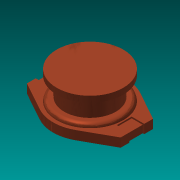
# Autodesk Inventor part: SDR1005
Saved by Autodesk Inventor 2015 (Build 190159000, 159)
## iProperties
Created: 2014-10-16
Part Number: SDR1005
Material: Generic
Document SubType Name: Modeling
Designer: Sawaiz Syed
Density: 1 g/cm^3
Appearance: Copper - Satin
Author: Sawaiz Syed
Autodesk Inventor part; units mm, degrees
ref_plane "YZ Plane" through (0, 0, 0) normal (1, 0, 0) x (0, 1, 0)
ref_plane "XZ Plane" through (0, 0, 0) normal (0, 1, 0) x (-1, 0, 0)
ref_plane "XY Plane" through (0, 0, 0) normal (0, 0, 1) x (1, 0, 0)
sketch "Sketch1" plane through (0, 0, 0) normal (0, 0, 1) x (1, 0, 0)
  line L0 (-6.35, 5) -> (6.35, 5)
  line L1 (6.35, 5) -> (6.35, -5)
  line L2 (6.35, -5) -> (-6.35, -5)
  line L3 (-6.35, -5) -> (-6.35, 5)
  line L4 (-6.35, 5) -> (6.35, -5) construction
  line L5 (6.35, 5) -> (-6.35, -5) construction
  line L6 (-2.4214, 4.3746) -> (-6.35, 2.2)
  line L7 (-2.4214, -4.3746) -> (-6.35, -2.2)
  line L8 (0, -5) -> (0, 5)
  line L9 (2.4214, 4.3746) -> (6.35, 2.2)
  line L10 (2.4214, -4.3746) -> (6.35, -2.2)
  line L11 (-6.35, 2.2) -> (-6.35, -2.2)
  line L12 (6.35, -2.2) -> (6.35, 2.2)
  arc A0 (-2.4214, -4.3746) -> (2.4214, -4.3746) centre (0, 0) ccw
  arc A1 (2.4214, 4.3746) -> (-2.4214, 4.3746) centre (0, 0) ccw
  point P0 (-1.2915, 5)
  point P1 (-1.2915, -5)
  point P2 (1.2915, 5)
  point P3 (1.2915, -5)
  dimension "d0" = 12.7
  dimension "d1" = 10
  dimension "d3" = 2.8
  dimension "d4" = 2.8
  constraints: 26 end point, 6 point on circle, 4 midpoint, 4 point on line, 4 symmetric about line, 3 tangent, 2 centre point, 2 collinear, 2 parallel, 1 coincident, 1 horizontal, 1 perpendicular
  measures "d0" distance of L1.end L2.end
  measures "d1" distance of L0.end L1.end
  measures "d3" distance of L0.start L6.end
  measures "d4" distance of L2.end L7.end
extrude "Extrusion1" add sketch "Sketch1" along normal blind 1.2 contours A1 L9 L1 L10 A0 L8 | L8 A0 L7 L3 L6 A1
sketch "Sketch2" plane through (0, 0, 1.2) normal (0, 0, 1) x (1, 0, 0)
  arc A0 (2.4214, 4.3746) -> (-2.4214, 4.3746) centre (0, 0) ccw projected
  circle A1 centre (0, 0) radius 3.5
  circle A2 centre (0, 0) radius 4.5
  dimension "d7" = 7
  dimension "d8" = 1
  constraints: 2 centre point, 1 coincident
  measures "d7" diameter of A1
  measures "d8" radial gap between concentric circles of A1 A2
extrude "Extrusion2" add sketch "Sketch2" along normal blind 0.5 contours A1 | A2
sketch "Sketch3" plane through (0, 0, 1.7) normal (0, 0, 1) x (1, 0, 0)
  circle A0 centre (0, 0) radius 4.5 projected
  circle A1 centre (0, 0) radius 3.5
  dimension "d11" = 7
  constraints: 1 centre point, 1 coincident
  measures "d11" diameter of A1
extrude "Extrusion3" add sketch "Sketch3" along normal blind 2.5 contours A1
sketch "Sketch4" plane through (0, 0, 4.2) normal (0, 0, 1) x (1, 0, 0)
  circle A0 centre (0, 0) radius 4.5
  dimension "d14" = 9
  constraints: 1 centre point, 1 coincident
  measures "d14" diameter of A0
extrude "Extrusion4" add sketch "Sketch4" along normal blind 0.8
fillet "Fillet1" radius 0.5 1 edges at (-4.5, 0, 1.7)
sketch "Sketch5" plane through (0, 0, 1.2) normal (0, 0, 1) x (1, 0, 0)
  circle A0 centre (0, 0) radius 4.5 projected
  line L0 (-6.35, 2.2) -> (-6.35, -2.2) projected
  line L1 (-6.35, -2.2) -> (-2.4214, -4.3746) projected
  arc A1 (-2.4214, -4.3746) -> (2.4214, -4.3746) centre (0, 0) ccw projected
  line L2 (2.4214, -4.3746) -> (6.35, -2.2) projected
  line L3 (6.35, -2.2) -> (6.35, 2.2) projected
  line L4 (6.35, 2.2) -> (2.4214, 4.3746) projected
  arc A2 (2.4214, 4.3746) -> (-2.4214, 4.3746) centre (0, 0) ccw projected
  line L5 (-2.4214, 4.3746) -> (-6.35, 2.2) projected
  line L6 (-6.35, 2.2) -> (-6.35, -2.2) projected
  line L7 (-6.35, 1) -> (-6.15, 1)
  line L8 (-6.15, 1) -> (-6.15, -1)
  line L9 (-6.15, -1) -> (-6.35, -1)
  line L10 (-6.35, -1) -> (-6.35, 1)
  line L11 (6.35, -1) -> (6.15, -1)
  line L12 (6.15, -1) -> (6.15, 1)
  line L13 (6.15, 1) -> (6.35, 1)
  line L14 (6.35, 1) -> (6.35, -1)
  point P0 (6.35, 0)
  point P1 (-6.35, 0)
  dimension "d18" = 2
  dimension "d19" = 2
  dimension "d20" = 0.2
  dimension "d21" = 0.2
  constraints: 16 end point, 4 midpoint, 4 parallel, 2 horizontal, 2 perpendicular, 2 point on line
  measures "d18" distance of L7.end L8.end
  measures "d19" distance of L11.end L12.end
  measures "d20" distance of L8.end L9.end
  measures "d21" distance of L11.start L11.end
extrude "Extrusion5" cut sketch "Sketch5" against normal through all contours L7 L8 L9 L0 | L3 L11 L12 L13
sketch "Sketch6" plane through (0, 0, 1.2) normal (0, 0, 1) x (1, 0, 0)
  line L0 (-6.15, -1) -> (-6.35, -1) projected
  line L1 (-6.35, -1) -> (-6.35, -2.2) projected
  line L2 (-6.35, -2.2) -> (-2.4214, -4.3746) projected
  arc A0 (-2.4214, -4.3746) -> (2.4214, -4.3746) centre (0, 0) ccw projected
  line L3 (2.4214, -4.3746) -> (6.35, -2.2) projected
  line L4 (6.35, -2.2) -> (6.35, -1) projected
  line L5 (6.35, -1) -> (6.15, -1) projected
  line L6 (6.15, -1) -> (6.15, 1) projected
  line L7 (6.15, 1) -> (6.35, 1) projected
  line L8 (6.35, 1) -> (6.35, 2.2) projected
  line L9 (6.35, 2.2) -> (2.4214, 4.3746) projected
  arc A1 (2.4214, 4.3746) -> (-2.4214, 4.3746) centre (0, 0) ccw projected
  line L10 (-2.4214, 4.3746) -> (-6.35, 2.2) projected
  line L11 (-6.35, 2.2) -> (-6.35, 1) projected
  line L12 (-6.35, 1) -> (-6.15, 1) projected
  line L13 (-6.15, 1) -> (-6.15, -1) projected
  circle A2 centre (0, 0) radius 4.5 projected
  line L14 (-6.15, 1) -> (-4.65, 1)
  line L15 (-4.65, 1) -> (-4.65, -1)
  line L16 (-4.65, -1) -> (-6.15, -1)
  line L17 (-6.15, -1) -> (-6.15, 1)
  line L18 (6.15, -1) -> (4.65, -1)
  line L19 (4.65, -1) -> (4.65, 1)
  line L20 (4.65, 1) -> (6.15, 1)
  line L21 (6.15, 1) -> (6.15, -1)
  dimension "d24" = 1.5
  dimension "d25" = 1.5
  constraints: 16 end point, 4 parallel, 2 horizontal, 2 perpendicular
  measures "d24" distance of L5.end L18.end
  measures "d25" distance of L15.end L16.end
extrude "Extrusion6" cut sketch "Sketch6" against normal blind 0.2 contours L13 L14 L15 L16 | L18 L19 L20 L6
body "Solid1"
